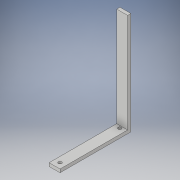
# Autodesk Inventor part: piezasoportepantalla
Saved by Autodesk Inventor 2019 (Build 230136000, 136)
## iProperties
Created: 2019-03-07
Part Number: piezasoportepantalla
Material: Genérico
Document SubType Name: Modeling
Designer: flakt
Density: 1 g/cm^3
Appearance: Valor por defecto
Author: flakt
Autodesk Inventor part; units mm, degrees
ref_plane "YZ Plane" through (0, 0, 0) normal (1, 0, 0) x (0, 1, 0)
ref_plane "XZ Plane" through (0, 0, 0) normal (0, 1, 0) x (-1, 0, 0)
ref_plane "XY Plane" through (0, 0, 0) normal (0, 0, 1) x (1, 0, 0)
sketch "Boceto1" plane through (0, 0, 0) normal (0, 1, 0) x (-1, 0, 0)
  circle A0 centre (20.1414, -70.1386) radius 1.5
  circle A1 centre (20.1414, -15.4215) radius 1.5
  line L0 (115.646, -75.4125) -> (-5.464, -75.4125)
  line L1 (20.1414, -75.4125) -> (15.1414, -75.4125)
  line L2 (15.1414, -75.4125) -> (25.1414, -75.4125)
  line L3 (25.1414, -75.4125) -> (25.1414, -10.4125)
  line L4 (25.1414, -10.4125) -> (15.1414, -10.4125)
  line L5 (15.1414, -10.4125) -> (15.1414, -75.4125)
  circle A2 centre (20.1414, -70.1386) radius 1.5
  circle A3 centre (20.1414, -15.4215) radius 1.5
  line L6 (115.646, -75.4125) -> (-5.464, -75.4125)
  line L7 (20.1414, -75.4125) -> (15.1414, -75.4125)
  line L8 (15.1414, -75.4125) -> (25.1414, -75.4125)
  line L9 (25.1414, -75.4125) -> (25.1414, -10.4125)
  line L10 (25.1414, -10.4125) -> (15.1414, -10.4125)
  line L11 (15.1414, -10.4125) -> (15.1414, -75.4125)
  point P0 (0, 0)
  dimension "d0" = 5
  dimension "d1" = 10
  dimension "d2" = 65
  dimension "d3" = 5
  dimension "d4" = 10
  dimension "d5" = 65
  constraints: 24 end point, 4 centre point, 4 parallel, 4 point on line, 2 horizontal, 2 perpendicular
  measures "d0" distance of L1.start L1.end
  measures "d1" distance of L4.end L3.end
  measures "d2" distance of L3.end L2.end
  measures "d3" distance of L7.start L7.end
  measures "d4" distance of L10.end L9.end
  measures "d5" distance of L9.end L8.end
extrude "Extrusión1" add sketch "Boceto1" along normal blind 3
sketch "Boceto2" plane through (0, 3, 0) normal (0, 1, 0) x (1, 0, 0)
  line L0 (-15.1414, 75.4125) -> (-25.1414, 75.4125) projected
  line L1 (-15.1414, 10.4125) -> (-15.1414, 75.4125) projected
  line L2 (-25.1414, 75.4125) -> (-15.1414, 75.4125)
  line L3 (-15.1414, 75.4125) -> (-15.1414, 72.4125)
  line L4 (-15.1414, 72.4125) -> (-25.1414, 72.4125)
  line L5 (-25.1414, 72.4125) -> (-25.1414, 75.4125)
  point P0 (0, 0)
  dimension "d8" = 3
  constraints: 8 end point, 2 parallel, 1 horizontal, 1 perpendicular, 1 point on line
  measures "d8" distance of L2.end L3.end
extrude "Extrusión2" add sketch "Boceto2" along normal blind 91
